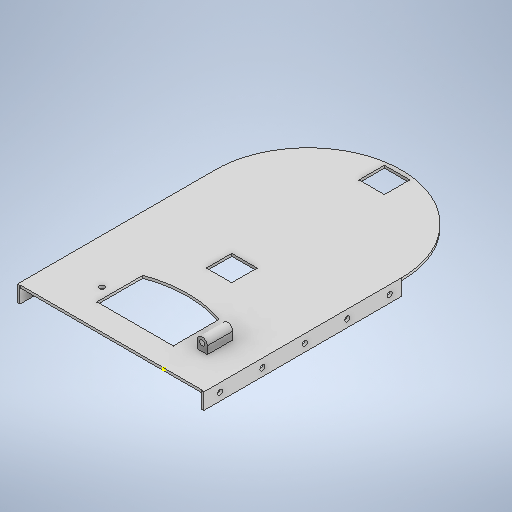
# Autodesk Inventor part: 1 part 07
Saved by Autodesk Inventor 2025.1 (Build 291241000, 241)
## iProperties
Created: 2024-07-30
Part Number: 1 part 07
Material: Generic
Document SubType Name: Modeling
Designer: Fabri
Density: 1 g/cm^3
Appearance: Default
Author: Fabri
Autodesk Inventor part; units mm, degrees
ref_plane "XZ Plane" through (0, 0, 0) normal (0, 1, 0) x (-1, 0, 0)
ref_plane "XY Plane" through (0, 0, 0) normal (0, 0, 1) x (1, 0, 0)
sketch "Sketch2" plane through (0, 0, 0) normal (0, 0, 1) x (1, 0, 0)
  line L0 (-55, 0) -> (55, 0)
  line L1 (55, 0) -> (55, 116)
  arc A0 (55, 116) -> (-55, 116) centre (0, 116) ccw
  line L2 (-55, 116) -> (-55, 0)
  point P0 (0, 0)
  point P1 (0, 0)
  dimension "d0" = 55
  dimension "d1" = 116
  constraints: 7 end point, 2 perpendicular, 2 point on circle, 1 centre point, 1 coincident, 1 horizontal, 1 horizontal alignment, 1 midpoint, 1 tangent
  measures "d0" radius of A0
  measures "d1" distance from line of L0 A0.centre
extrude "Extrusion1" add sketch "Sketch2" along normal mid plane 1.5
sketch "Sketch3" plane through (0, 0, 0.75) normal (0, 0, 1) x (1, 0, 0)
  line L0 (-22.5, 14) -> (22.5, 14)
  line L1 (22.5, 14) -> (22.5, 40.9816)
  line L2 (-22.5, 40.9816) -> (-22.5, 14)
  arc A0 (22.5, 40.9816) -> (-22.5, 40.9816) centre (0, -20) ccw
  arc A1 (55, 116) -> (-55, 116) centre (0, 116) ccw projected
  line L3 (-55, 0) -> (55, 0) projected
  point P0 (0, 0)
  point P1 (0, 14)
  point P2 (0, 171)
  point P3 (0, 45)
  dimension "d4" = 65
  dimension "d5" = 45
  dimension "d6" = 14
  dimension "d7" = 31
  constraints: 6 end point, 4 point on circle, 2 vertical alignment, 1 centre point, 1 horizontal, 1 midpoint, 1 parallel, 1 perpendicular
  measures "d4" radius of A0
  measures "d5" distance between parallel lines of L1 L2
  measures "d6" distance between parallel lines of L3 L0
  measures "d7" distance of point (0, 14) point (0, 45)
extrude "Extrusion2" cut sketch "Sketch3" against normal up to surface (1.5 mm away)
sketch "Sketch4" plane through (0, 0, 0.75) normal (0, 0, 1) x (1, 0, 0)
  line L0 (-7.5, 63.5) -> (7.5, 63.5)
  line L1 (7.5, 63.5) -> (7.5, 78.5)
  line L2 (7.5, 78.5) -> (-7.5, 78.5)
  line L3 (-7.5, 78.5) -> (-7.5, 63.5)
  line L4 (-7.5, 153.5) -> (7.5, 153.5)
  line L5 (7.5, 153.5) -> (7.5, 168.5)
  line L6 (7.5, 168.5) -> (-7.5, 168.5)
  line L7 (-7.5, 168.5) -> (-7.5, 153.5)
  arc A0 (22.5, 40.9816) -> (-22.5, 40.9816) centre (0, -20) ccw projected
  arc A1 (55, 116) -> (-55, 116) centre (0, 116) ccw projected
  point P0 (0, 0)
  point P1 (0, 153.5)
  point P2 (0, 45)
  point P3 (0, 63.5)
  point P4 (0, 45)
  point P5 (7.5, 71)
  dimension "d10" = 15
  dimension "d11" = 15
  dimension "d12" = 15
  dimension "d13" = 15
  dimension "d14" = 37.5
  dimension "d15" = 37.5
  constraints: 16 end point, 4 parallel, 3 midpoint, 2 horizontal, 2 perpendicular, 2 point on circle, 2 vertical alignment
  measures "d10" distance between parallel lines of L5 L7
  measures "d11" distance between parallel lines of L4 L6
  measures "d12" distance between parallel lines of L0 L2
  measures "d13" distance from line of point (7.5, 71) L3
  measures "d14" distance from line of L2 A1.centre
  measures "d15" distance from line of A1.centre L4
extrude "Extrusion3" cut sketch "Sketch4" against normal up to surface (1.5 mm away)
sketch "Sketch6" plane through (55, 0, 0.75) normal (1, 0, 0) x (0, 0, -1)
  line L0 (0, 0) -> (0, 116) projected
  line L1 (1.5, 116) -> (0, 116) projected
  line L2 (1.5, 116) -> (1.5, 0) projected
  line L3 (0, 0) -> (1.5, 0) projected
  line L4 (0, -0.3907) -> (9.5, -0.3907)
  line L5 (9.5, -0.3907) -> (9.5, 116)
  line L6 (9.5, 116) -> (0, 116)
  line L7 (0, 116) -> (0, -0.3907)
  point P0 (0.75, 0)
  dimension "d18" = 9.5
  constraints: 8 end point, 2 parallel, 1 horizontal, 1 perpendicular
  measures "d18" distance between parallel lines of L5 L0
extrude "Extrusion4" add sketch "Sketch6" against normal blind 1.5
sketch "Sketch7" plane through (55, -0.3907, 0.75) normal (1, 0, 0) x (0, 0, -1)
  line L0 (0, 0) -> (9.5, 0) projected
  line L1 (0, 116.3907) -> (0, 0) projected
  point P0 (0.75, 0.3907)
  point P1 (5, 109.5)
  point P2 (5, 84.5)
  point P3 (5, 59.5)
  point P4 (5, 34.5)
  point P5 (5, 9.5)
  dimension "d21" = 9.5
  dimension "d22" = 25
  dimension "d23" = 25
  dimension "d24" = 25
  dimension "d25" = 25
  dimension "d26" = 5
  constraints: 4 vertical alignment
  measures "d21" distance from line of L0 point (5, 9.5)
  measures "d22" distance of point (5, 9.5) point (5, 34.5)
  measures "d23" distance of point (5, 34.5) point (5, 59.5)
  measures "d24" distance of point (5, 59.5) point (5, 84.5)
  measures "d25" distance of point (5, 84.5) point (5, 109.5)
  measures "d26" distance from line of L1 point (5, 109.5)
hole "Hole1" at (55, 109.1093, -4.25) at (55, 84.1093, -4.25) at (55, 59.1093, -4.25) at (55, 34.1093, -4.25) at (55, 9.1093, -4.25) direction (-1, 0, 0) diameter 3 depth 1.5
mirror "Mirror1" about plane through (0, 0, 0) normal (1, 0, 0) of "Extrusion4", "Hole1"
ref_plane "Work Plane1" through (31, 0, 0) normal (1, 0, 0) x (0, 1, 0)
sketch "Sketch8" plane through (31, 0, 0) normal (1, 0, 0) x (0, 1, 0)
  point P0 (0, 0)
sketch "Sketch9" plane through (31, 0, 0) normal (1, 0, 0) x (0, 1, 0)
  line L0 (40.9816, 0.75) -> (14, 0.75) projected
  line L1 (14, 0.75) -> (40.9816, 0.75) projected
  line L2 (34.6093, 0.75) -> (34.6093, 5.25)
  line L3 (34.6093, 5.25) -> (19.6093, 5.25)
  line L4 (19.6093, 5.25) -> (19.6093, 0.75)
  line L5 (-0.3907, -8.75) -> (-0.3907, 0.75) projected
  point P0 (0, 0)
  dimension "d35" = 20
  dimension "d36" = 15
  dimension "d37" = 4.5
  constraints: 6 end point, 2 point on line, 1 parallel, 1 perpendicular, 1 vertical
  measures "d35" distance between parallel lines of L5 L4
  measures "d36" distance between parallel lines of L4 L2
  measures "d37" distance between parallel lines of L0 L3
extrude "Extrusion5" add sketch "Sketch9" along normal blind 6
sketch "Sketch10" plane through (31, 34.6093, 5.25) normal (0, 1, 0) x (1, 0, 0)
  line L0 (0, 4.5) -> (0, 0) projected
  line L1 (0, 0) -> (6, 0) projected
  line L2 (6, 4.5) -> (6, 0) projected
  line L3 (0, 4.5) -> (6, 4.5) projected
  arc A0 (0, 0) -> (6, 0) centre (3, 0) ccw
  point P0 (-31, 5.25)
  constraints: 2 point on circle, 2 tangent, 1 centre point
extrude "Extrusion6" add sketch "Sketch10" against normal up to surface (15 mm away) contours L1 A0
sketch "Sketch11" plane through (31, 19.6093, 0.75) normal (0, -1, 0) x (1, 0, 0)
  arc A0 (6, 4.5) -> (0, 4.5) centre (3, 4.5) ccw projected
  point P0 (-31, -0.75)
  point P1 (3, 7.5)
  constraints: 1 coincident, 1 point on circle, 1 vertical alignment
hole "Hole2" at (34, 19.6093, 5.25) direction (0, 1, 0) diameter 3 depth 15
sketch "Sketch12" plane through (0, 0, 0.75) normal (0, 0, 1) x (1, 0, 0)
  circle A0 centre (-28.5, 23) radius 1.5
  line L0 (-22.5, 14) -> (-22.5, 40.9816) projected
  line L1 (-53.5, 0) -> (53.5, 0) projected
  point P0 (0, 0)
  dimension "d49" = 3
  dimension "d50" = 6
  dimension "d51" = 23
  constraints: 1 centre point
  measures "d49" diameter of A0
  measures "d50" distance from line of L0 A0.centre
  measures "d51" distance from line of L1 A0.centre
extrude "Extrusion7" cut sketch "Sketch12" against normal up to surface (1.5 mm away)
equation "\"d13\" = d12"
equation "\"d15\" = d14"
equation "\"d23\" = d22"
equation "\"d24\" = d22"
equation "\"d25\" = d22"
body "Solid1"
